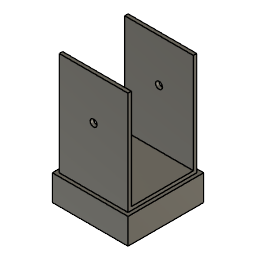
Moving Head (Autodesk Fusion 360 design; units mm, degrees)
Autodesk Fusion 360 part; units mm, degrees
sketch "Sketch1" plane through (0, 0, 0) normal (0, 0, 1) x (1, 0, 0) in component "Base housing"
  line L0 (21, 21) -> (-21, 21)
  line L1 (-21, 21) -> (-21, -21)
  line L2 (-21, -21) -> (21, -21)
  line L3 (21, -21) -> (21, 21)
  line L4 (21, 21) -> (-21, -21) construction
  line L5 (-21, 21) -> (21, -21) construction
  line L6 (22, 22) -> (-22, 22)
  line L7 (-22, 22) -> (-22, -22)
  line L8 (-22, -22) -> (22, -22)
  line L9 (22, -22) -> (22, 22)
  line L10 (22, 22) -> (-22, -22) construction
  line L11 (-22, 22) -> (22, -22) construction
  circle A0 centre (0, 0) radius 2
  dimension "d1" = 42
  dimension "d2" = 42
  dimension "d3" = 44
  dimension "d4" = 44
  dimension "d5" = 4
  constraint horizontal L0
  constraint perpendicular L0 L1
  constraint parallel L0 L2
  constraint parallel L1 L3
  constraint coincident L4 A0.centre
  constraint coincident L5 A0.centre
  constraint coincident A0.centre origin
  constraint horizontal L6
  constraint perpendicular L6 L7
  constraint parallel L6 L8
  constraint parallel L7 L9
  constraint coincident L10 A0.centre
  constraint coincident L11 A0.centre
  measures "d1" distance of L1.end L2.end
  measures "d2" distance of L0.end L1.end
  measures "d3" distance of L7.end L8.end
  measures "d4" distance of L6.end L7.end
  measures "d5" diameter of A0
extrude "Extrude1" add sketch "Sketch1" along normal blind 15 contours L0 L1 L2 L3 | L6 L7 L8 L9 makes body 1 in component "Base housing"
extrude "Extrude2" cut sketch "Sketch1" along normal blind 12 contours L0 L1 L2 L3 bodies 1 in component "Base housing"
sketch "Sketch1 (2)" plane through (-22, 0, 0) normal (-1, 0, 0) x (0, -1, 0) in component "Tilt mount"
  line L0 (-22, 0) -> (22, 0)
  line L1 (22, 0) -> (22, 15)
  line L2 (22, 15) -> (-22, 15)
  line L3 (-22, 15) -> (-22, 0)
  line L4 (-20, 15) -> (20, 15)
  line L5 (20, 15) -> (20, 75)
  line L6 (20, 75) -> (-20, 75)
  line L7 (-20, 75) -> (-20, 15)
  line L8 (-18, 75) -> (18, 75)
  line L9 (18, 75) -> (18, 17)
  line L10 (18, 17) -> (-18, 17)
  line L11 (-18, 17) -> (-18, 75)
  dimension "d10" = 40
  dimension "d11" = 60
  dimension "d12" = 36
  dimension "d13" = 58
  constraint horizontal L4
  constraint vertical L5
  constraint horizontal L6
  constraint vertical L7
  constraint coincident L2 L4.start
  constraint horizontal L8
  constraint vertical L9
  constraint horizontal L10
  constraint vertical L11
  constraint coincident L6 L8.start
  measures "d10" distance of L4.start L4.end
  measures "d11" distance of L4.start L6.end
  measures "d12" distance of L8.start L8.end
  measures "d13" distance of L8.start L10.end
extrude "Extrude1'" add sketch "Sketch1 (2)" along normal mid plane 40 from surface at -22 separate body contours L2 L4 L5 L6 L7 L9 L10 L11 makes body 2 in component "Tilt mount"
sketch "Sketch2" plane through (0, -22, 0) normal (0, -1, 0) x (1, 0, 0) in component "Tilt mount"
  line L0 (-22, 0) -> (22, 0)
  line L1 (22, 0) -> (22, 15)
  line L2 (22, 15) -> (-22, 15)
  line L3 (-22, 15) -> (-22, 0)
  line L4 (0, 75) -> (0, 70) construction
  line L5 (0, 70) -> (0, 50) construction
  circle A0 centre (0, 50) radius 2
  dimension "d17" = 5
  dimension "d18" = 20
  dimension "d19" = 4
  constraint vertical L4
  constraint parallel L4 L5
  constraint coincident L5.end A0.centre
  measures "d17" distance of L4.start L4.end
  measures "d18" distance of L4.end L5.end
  measures "d19" diameter of A0
extrude "Extrude2'" cut sketch "Sketch2" against normal blind 44 contours A0 bodies 2 in component "Tilt mount"
component "Base housing" placed x (1, 0, 0) y (0, 1, 0) z (0, 0, 1) at (0, 0, 0)
component "Tilt mount" placed x (1, 0, 0) y (0, 1, 0) z (0, 0, 1) at (0, 0, 0)
